Autodesk Fusion 360 part; units mm, degrees
(part 2 of 2)
  spline S369 degree 3 poles (-15.1942, 11.595) (-14.4543, 12.2873) (-14.1797, 12.9796) (-14.2633, 13.9224) knots 0 0 0 0 1 1 1 1
  spline S370 degree 3 poles (-14.2633, 13.9224) (-14.3946, 15.3547) (-15.6001, 16.4289) (-17.092, 16.4289) knots 0 0 0 0 1 1 1 1
  spline S371 degree 3 poles (-17.092, 16.4289) (-17.6291, 16.4289) (-18.7749, 15.7844) (-19.0733, 15.3189) knots 0 0 0 0 1 1 1 1
  spline S372 degree 3 poles (-19.0733, 15.3189) (-20.1355, 13.6837) (-19.4433, 11.6309) (-17.641, 11.058) knots 0 0 0 0 1 1 1 1
  spline S373 degree 3 poles (-17.641, 11.058) (-16.7403, 10.8043) (-15.715, 11.0847) (-15.1942, 11.595) knots 0 0 0 0 1 1 1 1
  spline S374 degree 3 poles (-66.0987, 20.2601) (-65.6691, 20.8688) (-65.5974, 21.4298) (-65.8361, 22.3369) knots 0 0 0 0 1 1 1 1
  spline S375 degree 3 poles (-65.8361, 22.3369) (-66.2061, 23.805) (-66.9461, 27.6482) (-67.161, 29.3191) knots 0 0 0 0 1 1 1 1
  spline S376 degree 3 poles (-67.161, 29.3191) (-67.2923, 30.2859) (-67.4474, 30.632) (-67.7577, 30.632) knots 0 0 0 0 1 1 1 1
  spline S377 degree 3 poles (-67.7577, 30.632) (-68.4142, 30.632) (-69.2497, 29.4265) (-69.2497, 28.4717) knots 0 0 0 0 1 1 1 1
  spline S378 degree 3 poles (-69.2497, 28.4717) (-69.2497, 27.9107) (-68.7364, 24.4733) (-68.5335, 23.5901) knots 0 0 0 0 1 1 1 1
  spline S379 degree 3 poles (-68.5335, 23.5901) (-68.3426, 22.8024) (-67.9368, 21.2388) (-67.7458, 20.5108) knots 0 0 0 0 1 1 1 1
  spline S380 degree 3 poles (-67.7458, 20.5108) (-67.6503, 20.1647) (-67.4594, 19.7708) (-67.3281, 19.6395) knots 0 0 0 0 1 1 1 1
  spline S381 degree 3 poles (-67.3281, 19.6395) (-67.1013, 19.4127) (-67.0774, 19.4127) (-66.7671, 19.5918) knots 0 0 0 0 1 1 1 1
  spline S382 degree 3 poles (-66.7671, 19.5918) (-66.5881, 19.6992) (-66.2897, 19.9976) (-66.0987, 20.2601) knots 0 0 0 0 1 1 1 1
  spline S383 degree 3 poles (-58.9494, 26.2159) (-58.0185, 26.3591) (-57.6127, 26.5978) (-57.4336, 27.123) knots 0 0 0 0 1 1 1 1
  spline S384 degree 3 poles (-57.4336, 27.123) (-57.171, 27.8988) (-57.5291, 28.2688) (-59.3314, 29.0685) knots 0 0 0 0 1 1 1 1
  spline S385 degree 3 poles (-59.3314, 29.0685) (-60.6084, 29.6294) (-60.9426, 29.6652) (-61.4917, 29.2833) knots 0 0 0 0 1 1 1 1
  spline S386 degree 3 poles (-61.4917, 29.2833) (-62.0884, 28.8894) (-62.351, 28.4478) (-62.4226, 27.7794) knots 0 0 0 0 1 1 1 1
  spline S387 degree 3 poles (-62.4226, 27.7794) (-62.4823, 27.0753) (-62.16, 26.4307) (-61.6349, 26.2278) knots 0 0 0 0 1 1 1 1
  spline S388 degree 3 poles (-61.6349, 26.2278) (-61.2171, 26.0727) (-59.9639, 26.0727) (-58.9494, 26.2159) knots 0 0 0 0 1 1 1 1
  spline S389 degree 3 poles (-19.3597, 26.3353) (-15.8984, 26.4427) (-15.0868, 26.5501) (-13.4159, 27.123) knots 0 0 0 0 1 1 1 1
  spline S390 degree 3 poles (-13.4159, 27.123) (-5.6927, 30.0385) (-15.6264, 35.7741) (-17.5933, 36.9697) knots 0 0 0 0 1 1 1 1
  spline S391 degree 3 poles (-17.5933, 36.9697) (-17.8678, 37.1487) (-19.8371, 38.3542) (-21.9497, 39.6552) knots 0 0 0 0 1 1 1 1
  spline S392 degree 3 poles (-21.9497, 39.6552) (-24.0742, 40.9681) (-26.0793, 42.1974) (-26.4255, 42.4003) knots 0 0 0 0 1 1 1 1
  spline S393 degree 3 poles (-26.4255, 42.4003) (-26.7716, 42.6032) (-28.0725, 43.379) (-29.3019, 44.1309) knots 0 0 0 0 1 1 1 1
  spline S394 degree 3 poles (-29.3019, 44.1309) (-30.5312, 44.8829) (-31.7725, 45.6229) (-32.047, 45.778) knots 0 0 0 0 1 1 1 1
  spline S395 degree 3 poles (-32.047, 45.778) (-32.6557, 46.1122) (-33.6464, 46.6851) (-35.5441, 47.7951) knots 0 0 0 0 1 1 1 1
  spline S396 degree 3 poles (-35.5441, 47.7951) (-38.3745, 49.7231) (-42.4002, 49.8932) (-44.7821, 48.2009) knots 0 0 0 0 1 1 1 1
  spline S397 degree 3 poles (-44.7821, 48.2009) (-45.6415, 47.5683) (-48.1837, 44.8709) (-50.2127, 42.4361) knots 0 0 0 0 1 1 1 1
  spline S398 degree 3 poles (-50.2127, 42.4361) (-50.7617, 41.7677) (-52.6714, 39.2016) (-53.3756, 38.1513) knots 0 0 0 0 1 1 1 1
  spline S399 degree 3 poles (-53.3756, 38.1513) (-53.8053, 37.5307) (-54.1753, 36.9936) (-54.2111, 36.9578) knots 0 0 0 0 1 1 1 1
  spline S400 degree 3 poles (-54.2111, 36.9578) (-54.2469, 36.922) (-54.3424, 36.7668) (-54.4378, 36.5997) knots 0 0 0 0 1 1 1 1
  spline S401 degree 3 poles (-54.4378, 36.5997) (-54.5333, 36.4326) (-54.8436, 35.8955) (-55.1301, 35.4062) knots 0 0 0 0 1 1 1 1
  spline S402 degree 3 poles (-55.1301, 35.4062) (-55.9536, 33.95) (-56.073, 32.673) (-55.512, 31.2049) knots 0 0 0 0 1 1 1 1
  spline S403 degree 3 poles (-55.512, 31.2049) (-54.7243, 29.1281) (-52.5759, 28.0778) (-48.0047, 27.5407) knots 0 0 0 0 1 1 1 1
  spline S404 degree 3 poles (-48.0047, 27.5407) (-39.6499, 26.562) (-27.9413, 26.0607) (-19.3597, 26.3353) knots 0 0 0 0 1 1 1 1
  spline S405 degree 3 poles (-63.9742, 31.2407) (-63.3655, 31.563) (-62.8046, 32.4343) (-62.7807, 33.1026) knots 0 0 0 0 1 1 1 1
  spline S406 degree 3 poles (-62.7807, 33.1026) (-62.7568, 33.4607) (-62.9597, 39.1181) (-63.0791, 41.6723) knots 0 0 0 0 1 1 1 1
  spline S407 degree 3 poles (-63.0791, 41.6723) (-63.1029, 42.0781) (-63.1507, 42.1616) (-63.3775, 42.1855) knots 0 0 0 0 1 1 1 1
  spline S408 degree 3 poles (-63.3775, 42.1855) (-63.9384, 42.269) (-64.8216, 41.4097) (-65.0842, 40.5265) knots 0 0 0 0 1 1 1 1
  spline S409 degree 3 poles (-65.0842, 40.5265) (-65.4303, 39.3568) (-65.3349, 35.3465) (-64.8813, 32.6133) knots 0 0 0 0 1 1 1 1
  spline S410 degree 3 poles (-64.8813, 32.6133) (-64.6307, 31.1214) (-64.5113, 30.9543) (-63.9742, 31.2407) knots 0 0 0 0 1 1 1 1
  spline S411 degree 3 poles (-59.1046, 34.9287) (-58.8539, 34.9287) (-58.2691, 35.7284) (-58.1617, 36.2416) knots 0 0 0 0 1 1 1 1
  spline S412 degree 3 poles (-58.1617, 36.2416) (-58.102, 36.54) (-58.0185, 37.7574) (-57.9707, 38.9629) knots 0 0 0 0 1 1 1 1
  spline S413 degree 3 poles (-57.9707, 38.9629) (-55.0055, 52.9367) (-60.0287, 51.9617) (-60.0594, 39.8939) knots 0 0 0 0 1 1 1 1
  spline S414 degree 3 poles (-60.0594, 39.8939) (-60.0475, 35.6091) (-59.9162, 34.6662) (-59.3672, 34.8691) knots 0 0 0 0 1 1 1 1
  spline S415 degree 3 poles (-59.3672, 34.8691) (-59.2717, 34.9049) (-59.1523, 34.9287) (-59.1046, 34.9287) knots 0 0 0 0 1 1 1 1
  spline S416 degree 3 poles (-53.483, 42.8897) (-53.0295, 43.1642) (-52.8504, 43.6535) (-52.5401, 45.4916) knots 0 0 0 0 1 1 1 1
  spline S417 degree 3 poles (-52.5401, 45.4916) (-47.8194, 56.8739) (-51.9428, 63.1533) (-54.1514, 48.6187) knots 0 0 0 0 1 1 1 1
  spline S418 degree 3 poles (-54.1514, 48.6187) (-54.4975, 46.3032) (-54.7004, 43.3551) (-54.5572, 42.9493) knots 0 0 0 0 1 1 1 1
  spline S419 degree 3 poles (-54.5572, 42.9493) (-54.4378, 42.6271) (-53.9843, 42.6032) (-53.483, 42.8897) knots 0 0 0 0 1 1 1 1
sketch "Sketch3" plane through (0, 0, 0) normal (0, 1, 0) x (1, 0, 0)
  circle A0 centre (-16.9405, 13.7) radius 2.65
  line L0 (-24.8905, 7.37) -> (-22.6383, 9.3908)
  line L1 (-24.4945, 12.3026) -> (-27.2771, 11.1137)
  arc A1 (-27.2771, 11.1137) -> (-24.8905, 7.37) centre (-26.3931, 9.0447) ccw
  arc A2 (-22.6383, 9.3908) -> (-24.4945, 12.3026) centre (-23.807, 10.6933) ccw
  line L2 (-60.0053, 29.4008) -> (-57.9336, 28.3794)
  line L3 (-60.4832, 26.1063) -> (-58.2067, 26.4969)
  arc A3 (-58.2067, 26.4969) -> (-57.9336, 28.3794) centre (-58.3758, 27.4825) ccw
  arc A4 (-60.0053, 29.4008) -> (-60.4832, 26.1063) centre (-60.7791, 27.8311) ccw
  line L4 (-66.9923, 29.5599) -> (-65.485, 21.1385)
  line L5 (-69.4532, 29.1195) -> (-67.9459, 20.698)
  line L6 (-63.025, 16.5893) -> (-64.9793, 2.8727)
  line L7 (-58.3449, -1.6991) -> (-24.4432, 17.0672)
  line L8 (-25.5471, 21.7521) -> (-55.2793, 23.0246)
  arc A5 (-24.4432, 17.0672) -> (-25.5471, 21.7521) centre (-25.654, 19.2544) ccw
  arc A6 (-55.2793, 23.0246) -> (-63.025, 16.5893) centre (-55.6, 15.5314) ccw
  arc A7 (-64.9793, 2.8727) -> (-58.3449, -1.6991) centre (-60.5243, 2.2379) ccw
  arc A8 (-66.9923, 29.5599) -> (-69.4532, 29.1195) centre (-68.2228, 29.3397) ccw
  arc A9 (-67.9459, 20.698) -> (-65.485, 21.1385) centre (-66.7155, 20.9182) ccw
  line L9 (-14.8187, 9.7316) -> (-21.3854, 6.2205)
  line L10 (-18.1944, 18.2109) -> (-16.902, 18.1998)
  arc A10 (-14.8187, 9.7316) -> (-16.902, 18.1998) centre (-16.9405, 13.7) ccw
  line L11 (-59.106, -8.2167) -> (-32.5692, 5.579)
  line L12 (-29.2713, 2.0763) -> (-49.4618, -31.6353)
  line L13 (-57.5245, -30.9331) -> (-62.6501, -17.5544)
  line L14 (-70.8774, 23.2307) -> (-66.9031, 10.8336)
  line L15 (-73.2581, 22.4675) -> (-69.2838, 10.0704)
  line L16 (-68.0088, 1.6737) -> (-73.8434, 13.4497)
  line L17 (-76.0835, 12.3397) -> (-70.2489, 0.5638)
  line L18 (-74.8007, 3.5823) -> (-70.4064, -3.84)
  line L19 (-72.5576, -5.1137) -> (-76.9519, 2.3086)
  line L20 (-15.8372, -7.9675) -> (-16.0798, -15.41)
  arc A11 (-15.8372, -7.9675) -> (-24.2125, -5.5377) centre (-20.3348, -7.8209) ccw
  circle A12 centre (-20.3348, -7.8209) radius 2.65
  line L21 (-18.8278, -17.8708) -> (-19.4518, -14.9099)
  arc A13 (-19.4518, -14.9099) -> (-22.9016, -15.0616) centre (-21.1642, -15.2708) ccw
  line L22 (-22.9016, -15.0616) -> (-23.2633, -18.0658)
  arc A14 (-23.2633, -18.0658) -> (-18.8278, -17.8708) centre (-21.0294, -18.3348) ccw
  line L23 (-27.701, -51.3778) -> (-27.0022, -12.6349)
  arc A15 (-27.0022, -12.6349) -> (-31.6114, -11.2483) centre (-29.5018, -12.5898) ccw
  line L24 (-31.6114, -11.2483) -> (-47.5795, -36.361)
  arc A16 (-47.5795, -36.361) -> (-45.8793, -46.2866) centre (-41.2506, -40.3853) ccw
  line L25 (-45.8793, -46.2866) -> (-34.9774, -54.8374)
  arc A17 (-34.9774, -54.8374) -> (-27.701, -51.3778) centre (-32.2002, -51.2966) ccw
  line L26 (-1.0185, -17.6992) -> (5.3056, -21.6305)
  arc A18 (-1.0185, -17.6992) -> (-7.3105, -23.7375) centre (-3.3943, -21.5209) ccw
  circle A19 centre (-3.3943, -21.5209) radius 2.65
  line L27 (6.0627, -25.2408) -> (3.1865, -24.3007)
  arc A20 (3.1865, -24.3007) -> (1.5929, -27.3642) centre (2.6428, -25.9641) ccw
  line L28 (1.5929, -27.3642) -> (4.0138, -29.1795)
  arc A21 (4.0138, -29.1795) -> (6.0627, -25.2408) centre (5.3637, -27.3794) ccw
  line L29 (30.644, -49.6786) -> (-2.559, -29.702)
  arc A22 (-2.559, -29.702) -> (-6.0644, -33.0005) centre (-3.8478, -31.8442) ccw
  line L30 (-6.0644, -33.0005) -> (7.6998, -59.3856)
  arc A23 (7.6998, -59.3856) -> (17.1457, -62.8759) centre (14.3494, -55.9167) ccw
  line L31 (17.1457, -62.8759) -> (30.0019, -57.7101)
  arc A24 (30.0019, -57.7101) -> (30.644, -49.6786) centre (28.3241, -53.5345) ccw
  line L32 (14.8187, -9.7316) -> (21.3854, -6.2205)
  arc A25 (14.8187, -9.7316) -> (16.902, -18.1998) centre (16.9405, -13.7) ccw
  circle A26 centre (16.9405, -13.7) radius 2.65
  line L33 (24.8905, -7.37) -> (22.6383, -9.3908)
  arc A27 (22.6383, -9.3908) -> (24.4945, -12.3026) centre (23.807, -10.6933) ccw
  line L34 (24.4945, -12.3026) -> (27.2771, -11.1137)
  arc A28 (27.2771, -11.1137) -> (24.8905, -7.37) centre (26.3931, -9.0447) ccw
  line L35 (58.3449, 1.6991) -> (24.4432, -17.0672)
  arc A29 (24.4432, -17.0672) -> (25.5471, -21.7521) centre (25.654, -19.2544) ccw
  line L36 (25.5471, -21.7521) -> (55.2793, -23.0246)
  arc A30 (55.2793, -23.0246) -> (63.025, -16.5893) centre (55.6, -15.5314) ccw
  line L37 (63.025, -16.5893) -> (64.9793, -2.8727)
  arc A31 (64.9793, -2.8727) -> (58.3449, 1.6991) centre (60.5243, -2.2379) ccw
  line L38 (15.8372, 7.9675) -> (16.0798, 15.41)
  arc A32 (15.8372, 7.9675) -> (24.2125, 5.5377) centre (20.3348, 7.8209) ccw
  circle A33 centre (20.3348, 7.8209) radius 2.65
  line L39 (18.8278, 17.8708) -> (19.4518, 14.9099)
  arc A34 (19.4518, 14.9099) -> (22.9016, 15.0616) centre (21.1642, 15.2708) ccw
  line L40 (22.9016, 15.0616) -> (23.2633, 18.0658)
  arc A35 (23.2633, 18.0658) -> (18.8278, 17.8708) centre (21.0294, 18.3348) ccw
  line L41 (27.701, 51.3778) -> (27.0022, 12.6349)
  arc A36 (27.0022, 12.6349) -> (31.6114, 11.2483) centre (29.5018, 12.5898) ccw
  line L42 (31.6114, 11.2483) -> (47.5795, 36.361)
  arc A37 (47.5795, 36.361) -> (45.8793, 46.2866) centre (41.2506, 40.3853) ccw
  line L43 (45.8793, 46.2866) -> (34.9774, 54.8374)
  arc A38 (34.9774, 54.8374) -> (27.701, 51.3778) centre (32.2002, 51.2966) ccw
  line L44 (1.0185, 17.6992) -> (-5.3056, 21.6305)
  arc A39 (1.0185, 17.6992) -> (7.3105, 23.7375) centre (3.3943, 21.5209) ccw
  circle A40 centre (3.3943, 21.5209) radius 2.65
  line L45 (-6.0627, 25.2408) -> (-3.1865, 24.3007)
  arc A41 (-3.1865, 24.3007) -> (-1.5929, 27.3642) centre (-2.6428, 25.9641) ccw
  line L46 (-1.5929, 27.3642) -> (-4.0138, 29.1795)
  arc A42 (-4.0138, 29.1795) -> (-6.0627, 25.2408) centre (-5.3637, 27.3794) ccw
  line L47 (-30.644, 49.6786) -> (2.559, 29.702)
  arc A43 (2.559, 29.702) -> (6.0644, 33.0005) centre (3.8478, 31.8442) ccw
  line L48 (6.0644, 33.0005) -> (-7.6998, 59.3856)
  arc A44 (-7.6998, 59.3856) -> (-17.1457, 62.8759) centre (-14.3494, 55.9167) ccw
  line L49 (-17.1457, 62.8759) -> (-30.0019, 57.7101)
  arc A45 (-30.0019, 57.7101) -> (-30.644, 49.6786) centre (-28.3241, 53.5345) ccw
  arc A46 (-29.2713, 2.0763) -> (-32.5692, 5.579) centre (-31.4161, 3.3609) ccw
  arc A47 (-59.106, -8.2167) -> (-62.6501, -17.5544) centre (-55.6465, -14.8712) ccw
  arc A48 (-57.5245, -30.9331) -> (-49.4618, -31.6353) centre (-53.3224, -29.3232) ccw
  line L50 (-16.4338, -24.3115) -> (2.6661, -58.6528)
  arc A49 (-16.4338, -24.3115) -> (-21.1162, -25.4163) centre (-18.6186, -25.5267) ccw
  line L51 (-22.4371, -55.2957) -> (-21.1162, -25.4163)
  arc A50 (-22.4371, -55.2957) -> (-16.1225, -63.0338) centre (-14.9444, -55.6269) ccw
  line L52 (-1.9734, -65.2842) -> (-16.1225, -63.0338)
  arc A51 (-1.9734, -65.2842) -> (2.6661, -58.6528) centre (-1.2666, -60.8401) ccw
  line L53 (12.8375, -26.3878) -> (52.1279, -27.0175)
  arc A52 (12.8375, -26.3878) -> (11.453, -30.9953) centre (12.7974, -28.8875) ccw
  line L54 (36.6689, -47.0789) -> (11.453, -30.9953)
  arc A53 (36.6689, -47.0789) -> (46.5276, -45.4794) centre (40.7021, -40.7557) ccw
  line L55 (55.5511, -34.3512) -> (46.5276, -45.4794)
  arc A54 (55.5511, -34.3512) -> (52.1279, -27.0175) centre (52.0558, -31.5169) ccw
  line L56 (29.2713, -2.0763) -> (49.4618, 31.6353)
  arc A55 (29.2713, -2.0763) -> (32.5692, -5.579) centre (31.4161, -3.3609) ccw
  line L57 (59.106, 8.2167) -> (32.5692, -5.579)
  arc A56 (59.106, 8.2167) -> (62.6501, 17.5544) centre (55.6465, 14.8712) ccw
  line L58 (57.5245, 30.9331) -> (62.6501, 17.5544)
  arc A57 (57.5245, 30.9331) -> (49.4618, 31.6353) centre (53.3224, 29.3232) ccw
  line L59 (16.4338, 24.3115) -> (-2.6661, 58.6528)
  arc A58 (16.4338, 24.3115) -> (21.1162, 25.4163) centre (18.6186, 25.5267) ccw
  line L60 (22.4371, 55.2957) -> (21.1162, 25.4163)
  arc A59 (22.4371, 55.2957) -> (16.1225, 63.0338) centre (14.9444, 55.6269) ccw
  line L61 (1.9734, 65.2842) -> (16.1225, 63.0338)
  arc A60 (1.9734, 65.2842) -> (-2.6661, 58.6528) centre (1.2666, 60.8401) ccw
  line L62 (-12.8375, 26.3878) -> (-52.1279, 27.0175)
  arc A61 (-12.8375, 26.3878) -> (-11.453, 30.9953) centre (-12.7974, 28.8875) ccw
  line L63 (-36.6689, 47.0789) -> (-11.453, 30.9953)
  arc A62 (-36.6689, 47.0789) -> (-46.5276, 45.4794) centre (-40.7021, 40.7557) ccw
  line L64 (-55.5511, 34.3512) -> (-46.5276, 45.4794)
  arc A63 (-55.5511, 34.3512) -> (-52.1279, 27.0175) centre (-52.0558, 31.5169) ccw
  arc A64 (-70.8774, 23.2307) -> (-73.2581, 22.4675) centre (-72.0677, 22.8491) ccw
  arc A65 (-69.2838, 10.0704) -> (-66.9031, 10.8336) centre (-68.0934, 10.452) ccw
  arc A66 (-70.2489, 0.5638) -> (-68.0088, 1.6737) centre (-69.1288, 1.1187) ccw
  arc A67 (-73.8434, 13.4497) -> (-76.0835, 12.3397) centre (-74.9634, 12.8947) ccw
  arc A68 (-74.8007, 3.5823) -> (-76.9519, 2.3086) centre (-75.8763, 2.9454) ccw
  arc A69 (-72.5576, -5.1137) -> (-70.4064, -3.84) centre (-71.482, -4.4769) ccw
  line L65 (-18.3054, 22.707) -> (-11.1638, 23.121)
  line L66 (-28.8175, -4.4994) -> (-25.6053, 1.8924)
  line L67 (-10.5122, -27.2064) -> (-14.4415, -21.2286)
  line L68 (18.3054, -22.707) -> (11.1638, -23.121)
  line L69 (28.8175, 4.4994) -> (25.6053, -1.8924)
  line L70 (10.5122, 27.2064) -> (14.4415, 21.2286)
  line L71 (-24.8683, -6.6514) -> (-24.2125, -5.5377)
  line L72 (-6.6739, -24.8622) -> (-7.3105, -23.7375)
  line L73 (18.1944, -18.2109) -> (16.902, -18.1998)
  line L74 (24.8683, 6.6514) -> (24.2125, 5.5377)
  line L75 (6.6739, 24.8622) -> (7.3105, 23.7375)
  arc A70 (-18.3054, 22.707) -> (-18.1944, 18.2109) centre (-18.1752, 20.4608) ccw
  arc A71 (-5.3056, 21.6305) -> (-11.1638, 23.121) centre (-10.5851, 13.1378) ccw
  arc A72 (10.5122, 27.2064) -> (6.6739, 24.8622) centre (8.632, 25.9705) ccw
  arc A73 (16.0798, 15.41) -> (14.4415, 21.2286) centre (6.0851, 15.7358) ccw
  arc A74 (21.3854, -6.2205) -> (25.6053, -1.8924) centre (16.6702, 2.5981) ccw
  arc A75 (28.8175, 4.4994) -> (24.8683, 6.6514) centre (26.8071, 5.5098) ccw
  arc A76 (5.3056, -21.6305) -> (11.1638, -23.121) centre (10.5851, -13.1378) ccw
  arc A77 (18.3054, -22.707) -> (18.1944, -18.2109) centre (18.1752, -20.4608) ccw
  arc A78 (-16.0798, -15.41) -> (-14.4415, -21.2286) centre (-6.0851, -15.7358) ccw
  arc A79 (-10.5122, -27.2064) -> (-6.6739, -24.8622) centre (-8.632, -25.9705) ccw
  arc A80 (-21.3854, 6.2205) -> (-25.6053, 1.8924) centre (-16.6702, -2.5981) ccw
  arc A81 (-15.9874, -12.5747) -> (-15.5594, -12.5362) centre (-16.6702, -2.5981) ccw
  arc A82 (-28.8175, -4.4994) -> (-24.8683, -6.6514) centre (-26.8071, -5.5098) ccw
  line L76 (-66.6665, -4.5408) -> (-64.3617, -4.3895)
  arc A83 (-66.6665, -4.5408) -> (-65.4331, -7.6328) centre (-66.5518, -6.2871) ccw
  arc A84 (-63.6569, -6.1563) -> (-64.3617, -4.3895) centre (-64.2961, -5.3873) ccw
  line L77 (-65.4331, -7.6328) -> (-63.6569, -6.1563)
  arc A85 (-69.1919, -16.048) -> (-67.2809, -14.4361) centre (-68.2364, -15.242) ccw
  line L78 (-74.708, -9.5084) -> (-69.1919, -16.048)
  arc A86 (-72.797, -7.8965) -> (-74.708, -9.5084) centre (-73.7525, -8.7025) ccw
  line L79 (-72.797, -7.8965) -> (-67.2809, -14.4361)
  arc A87 (-65.0367, -25.9207) -> (-63.3566, -24.0694) centre (-64.1966, -24.9951) ccw
  line L80 (-74.6771, -17.1716) -> (-65.0367, -25.9207)
  arc A88 (-72.997, -15.3203) -> (-74.6771, -17.1716) centre (-73.837, -16.246) ccw
  line L81 (-72.997, -15.3203) -> (-63.3566, -24.0694)
  line L82 (-72.0601, -27.3552) -> (-61.1192, -34.6362)
  arc A89 (-61.1192, -34.6362) -> (-59.7342, -32.5549) centre (-60.4267, -33.5956) ccw
  arc A90 (-70.6751, -25.2739) -> (-72.0601, -27.3552) centre (-71.3676, -26.3146) ccw
  line L83 (-59.7342, -32.5549) -> (-70.6751, -25.2739)
  arc A91 (-60.2799, -40.7074) -> (-59.0537, -38.5288) centre (-59.6668, -39.6181) ccw
  line L84 (-60.2799, -40.7074) -> (-67.7966, -36.4766)
  arc A92 (-66.5704, -34.298) -> (-67.7966, -36.4766) centre (-67.1835, -35.3873) ccw
  line L85 (-66.5704, -34.298) -> (-59.0537, -38.5288)
  line L86 (-55.4644, -37.2657) -> (-53.5441, -35.9822)
  arc A93 (-55.4644, -37.2657) -> (-52.8503, -39.3268) centre (-54.492, -38.7207) ccw
  arc A94 (-52.0503, -37.16) -> (-53.5441, -35.9822) centre (-52.9884, -36.8136) ccw
  line L87 (-52.8503, -39.3268) -> (-52.0503, -37.16)
  arc A95 (-51.8979, -48.4939) -> (-51.0489, -46.1425) centre (-51.4734, -47.3182) ccw
  line L88 (-59.9448, -45.5885) -> (-51.8979, -48.4939)
  arc A96 (-59.0958, -43.2371) -> (-59.9448, -45.5885) centre (-59.5203, -44.4128) ccw
  line L89 (-59.0958, -43.2371) -> (-51.0489, -46.1425)
  arc A97 (-43.3631, -54.9663) -> (-42.8337, -52.523) centre (-43.0984, -53.7447) ccw
  line L90 (-56.0865, -52.2096) -> (-43.3631, -54.9663)
  arc A98 (-55.5571, -49.7663) -> (-56.0865, -52.2096) centre (-55.8218, -50.9879) ccw
  line L91 (-55.5571, -49.7663) -> (-42.8337, -52.523)
  line L92 (-48.7283, -59.7204) -> (-35.6127, -60.5554)
  arc A99 (-35.6127, -60.5554) -> (-35.4538, -58.0605) centre (-35.5333, -59.308) ccw
  arc A100 (-48.5694, -57.2254) -> (-48.7283, -59.7204) centre (-48.6489, -58.4729) ccw
  line L93 (-35.4538, -58.0605) -> (-48.5694, -57.2254)
  arc A101 (-31.8503, -65.3936) -> (-31.8776, -62.8937) centre (-31.8639, -64.1437) ccw
  line L94 (-31.8503, -65.3936) -> (-40.4753, -65.488)
  arc A102 (-40.5027, -62.9882) -> (-40.4753, -65.488) centre (-40.489, -64.2381) ccw
  line L95 (-40.5027, -62.9882) -> (-31.8776, -62.8937)
  line L96 (-29.4008, -60.0053) -> (-28.3794, -57.9336)
  arc A103 (-29.4008, -60.0053) -> (-26.1063, -60.4832) centre (-27.8311, -60.7791) ccw
  arc A104 (-26.4969, -58.2067) -> (-28.3794, -57.9336) centre (-27.4825, -58.3758) ccw
  line L97 (-26.1063, -60.4832) -> (-26.4969, -58.2067)
  arc A105 (-20.698, -67.9459) -> (-21.1385, -65.485) centre (-20.9182, -66.7155) ccw
  line L98 (-29.1195, -69.4532) -> (-20.698, -67.9459)
  arc A106 (-29.5599, -66.9923) -> (-29.1195, -69.4532) centre (-29.3397, -68.2228) ccw
  line L99 (-29.5599, -66.9923) -> (-21.1385, -65.485)
  arc A107 (-10.0704, -69.2838) -> (-10.8336, -66.9031) centre (-10.452, -68.0934) ccw
  line L100 (-22.4675, -73.2581) -> (-10.0704, -69.2838)
  arc A108 (-23.2307, -70.8774) -> (-22.4675, -73.2581) centre (-22.8491, -72.0677) ccw
  line L101 (-23.2307, -70.8774) -> (-10.8336, -66.9031)
  line L102 (-12.3397, -76.0835) -> (-0.5638, -70.2489)
  arc A109 (-0.5638, -70.2489) -> (-1.6737, -68.0088) centre (-1.1187, -69.1288) ccw
  arc A110 (-13.4497, -73.8434) -> (-12.3397, -76.0835) centre (-12.8947, -74.9634) ccw
  line L103 (-1.6737, -68.0088) -> (-13.4497, -73.8434)
  arc A111 (5.1137, -72.5576) -> (3.84, -70.4064) centre (4.4769, -71.482) ccw
  line L104 (5.1137, -72.5576) -> (-2.3086, -76.9519)
  arc A112 (-3.5823, -74.8007) -> (-2.3086, -76.9519) centre (-2.9454, -75.8763) ccw
  line L105 (-3.5823, -74.8007) -> (3.84, -70.4064)
  line L106 (4.5408, -66.6665) -> (4.3895, -64.3617)
  arc A113 (4.5408, -66.6665) -> (7.6328, -65.4331) centre (6.2871, -66.5518) ccw
  arc A114 (6.1563, -63.6569) -> (4.3895, -64.3617) centre (5.3873, -64.2961) ccw
  line L107 (7.6328, -65.4331) -> (6.1563, -63.6569)
  arc A115 (16.048, -69.1919) -> (14.4361, -67.2809) centre (15.242, -68.2364) ccw
  line L108 (9.5084, -74.708) -> (16.048, -69.1919)
  arc A116 (7.8965, -72.797) -> (9.5084, -74.708) centre (8.7025, -73.7525) ccw
  line L109 (7.8965, -72.797) -> (14.4361, -67.2809)
  arc A117 (25.9207, -65.0367) -> (24.0694, -63.3566) centre (24.9951, -64.1966) ccw
  line L110 (17.1716, -74.6771) -> (25.9207, -65.0367)
  arc A118 (15.3203, -72.997) -> (17.1716, -74.6771) centre (16.246, -73.837) ccw
  line L111 (15.3203, -72.997) -> (24.0694, -63.3566)
  line L112 (27.3552, -72.0601) -> (34.6362, -61.1192)
  arc A119 (34.6362, -61.1192) -> (32.5549, -59.7342) centre (33.5956, -60.4267) ccw
  arc A120 (25.2739, -70.6751) -> (27.3552, -72.0601) centre (26.3146, -71.3676) ccw
  line L113 (32.5549, -59.7342) -> (25.2739, -70.6751)
  arc A121 (40.7074, -60.2799) -> (38.5288, -59.0537) centre (39.6181, -59.6668) ccw
  line L114 (40.7074, -60.2799) -> (36.4766, -67.7966)
  arc A122 (34.298, -66.5704) -> (36.4766, -67.7966) centre (35.3873, -67.1835) ccw
  line L115 (34.298, -66.5704) -> (38.5288, -59.0537)
  line L116 (37.2657, -55.4644) -> (35.9822, -53.5441)
  arc A123 (37.2657, -55.4644) -> (39.3268, -52.8503) centre (38.7207, -54.492) ccw
  arc A124 (37.16, -52.0503) -> (35.9822, -53.5441) centre (36.8136, -52.9884) ccw
  line L117 (39.3268, -52.8503) -> (37.16, -52.0503)
  arc A125 (48.4939, -51.8979) -> (46.1425, -51.0489) centre (47.3182, -51.4734) ccw
  line L118 (45.5885, -59.9448) -> (48.4939, -51.8979)
  arc A126 (43.2371, -59.0958) -> (45.5885, -59.9448) centre (44.4128, -59.5203) ccw
  line L119 (43.2371, -59.0958) -> (46.1425, -51.0489)
  arc A127 (54.9663, -43.3631) -> (52.523, -42.8337) centre (53.7447, -43.0984) ccw
  line L120 (52.2096, -56.0865) -> (54.9663, -43.3631)
  arc A128 (49.7663, -55.5571) -> (52.2096, -56.0865) centre (50.9879, -55.8218) ccw
  line L121 (49.7663, -55.5571) -> (52.523, -42.8337)
  line L122 (59.7204, -48.7283) -> (60.5554, -35.6127)
  arc A129 (60.5554, -35.6127) -> (58.0605, -35.4538) centre (59.308, -35.5333) ccw
  arc A130 (57.2254, -48.5694) -> (59.7204, -48.7283) centre (58.4729, -48.6489) ccw
  line L123 (58.0605, -35.4538) -> (57.2254, -48.5694)
  arc A131 (65.3936, -31.8503) -> (62.8937, -31.8776) centre (64.1437, -31.8639) ccw
  line L124 (65.3936, -31.8503) -> (65.488, -40.4753)
  arc A132 (62.9882, -40.5027) -> (65.488, -40.4753) centre (64.2381, -40.489) ccw
  line L125 (62.9882, -40.5027) -> (62.8937, -31.8776)
  line L126 (60.0053, -29.4008) -> (57.9336, -28.3794)
  arc A133 (60.0053, -29.4008) -> (60.4832, -26.1063) centre (60.7791, -27.8311) ccw
  arc A134 (58.2067, -26.4969) -> (57.9336, -28.3794) centre (58.3758, -27.4825) ccw
  line L127 (60.4832, -26.1063) -> (58.2067, -26.4969)
  arc A135 (67.9459, -20.698) -> (65.485, -21.1385) centre (66.7155, -20.9182) ccw
  line L128 (69.4532, -29.1195) -> (67.9459, -20.698)
  arc A136 (66.9923, -29.5599) -> (69.4532, -29.1195) centre (68.2228, -29.3397) ccw
  line L129 (66.9923, -29.5599) -> (65.485, -21.1385)
  arc A137 (69.2838, -10.0704) -> (66.9031, -10.8336) centre (68.0934, -10.452) ccw
  line L130 (73.2581, -22.4675) -> (69.2838, -10.0704)
  arc A138 (70.8774, -23.2307) -> (73.2581, -22.4675) centre (72.0677, -22.8491) ccw
  line L131 (70.8774, -23.2307) -> (66.9031, -10.8336)
  line L132 (76.0835, -12.3397) -> (70.2489, -0.5638)
  arc A139 (70.2489, -0.5638) -> (68.0088, -1.6737) centre (69.1288, -1.1187) ccw
  arc A140 (73.8434, -13.4497) -> (76.0835, -12.3397) centre (74.9634, -12.8947) ccw
  line L133 (68.0088, -1.6737) -> (73.8434, -13.4497)
  arc A141 (72.5576, 5.1137) -> (70.4064, 3.84) centre (71.482, 4.4769) ccw
  line L134 (72.5576, 5.1137) -> (76.9519, -2.3086)
  arc A142 (74.8007, -3.5823) -> (76.9519, -2.3086) centre (75.8763, -2.9454) ccw
  line L135 (74.8007, -3.5823) -> (70.4064, 3.84)
  line L136 (66.6665, 4.5408) -> (64.3617, 4.3895)
  arc A143 (66.6665, 4.5408) -> (65.4331, 7.6328) centre (66.5518, 6.2871) ccw
  arc A144 (63.6569, 6.1563) -> (64.3617, 4.3895) centre (64.2961, 5.3873) ccw
  line L137 (65.4331, 7.6328) -> (63.6569, 6.1563)
  arc A145 (69.1919, 16.048) -> (67.2809, 14.4361) centre (68.2364, 15.242) ccw
  line L138 (74.708, 9.5084) -> (69.1919, 16.048)
  arc A146 (72.797, 7.8965) -> (74.708, 9.5084) centre (73.7525, 8.7025) ccw
  line L139 (72.797, 7.8965) -> (67.2809, 14.4361)
  arc A147 (65.0367, 25.9207) -> (63.3566, 24.0694) centre (64.1966, 24.9951) ccw
  line L140 (74.6771, 17.1716) -> (65.0367, 25.9207)
  arc A148 (72.997, 15.3203) -> (74.6771, 17.1716) centre (73.837, 16.246) ccw
  line L141 (72.997, 15.3203) -> (63.3566, 24.0694)
  line L142 (72.0601, 27.3552) -> (61.1192, 34.6362)
  arc A149 (61.1192, 34.6362) -> (59.7342, 32.5549) centre (60.4267, 33.5956) ccw
  arc A150 (70.6751, 25.2739) -> (72.0601, 27.3552) centre (71.3676, 26.3146) ccw
  line L143 (59.7342, 32.5549) -> (70.6751, 25.2739)
  arc A151 (60.2799, 40.7074) -> (59.0537, 38.5288) centre (59.6668, 39.6181) ccw
  line L144 (60.2799, 40.7074) -> (67.7966, 36.4766)
  arc A152 (66.5704, 34.298) -> (67.7966, 36.4766) centre (67.1835, 35.3873) ccw
  line L145 (66.5704, 34.298) -> (59.0537, 38.5288)
  line L146 (55.4644, 37.2657) -> (53.5441, 35.9822)
  arc A153 (55.4644, 37.2657) -> (52.8503, 39.3268) centre (54.492, 38.7207) ccw
  arc A154 (52.0503, 37.16) -> (53.5441, 35.9822) centre (52.9884, 36.8136) ccw
  line L147 (52.8503, 39.3268) -> (52.0503, 37.16)
  arc A155 (51.8979, 48.4939) -> (51.0489, 46.1425) centre (51.4734, 47.3182) ccw
  line L148 (59.9448, 45.5885) -> (51.8979, 48.4939)
  arc A156 (59.0958, 43.2371) -> (59.9448, 45.5885) centre (59.5203, 44.4128) ccw
  line L149 (59.0958, 43.2371) -> (51.0489, 46.1425)
  arc A157 (43.3631, 54.9663) -> (42.8337, 52.523) centre (43.0984, 53.7447) ccw
  line L150 (56.0865, 52.2096) -> (43.3631, 54.9663)
  arc A158 (55.5571, 49.7663) -> (56.0865, 52.2096) centre (55.8218, 50.9879) ccw
  line L151 (55.5571, 49.7663) -> (42.8337, 52.523)
  line L152 (48.7283, 59.7204) -> (35.6127, 60.5554)
  arc A159 (35.6127, 60.5554) -> (35.4538, 58.0605) centre (35.5333, 59.308) ccw
  arc A160 (48.5694, 57.2254) -> (48.7283, 59.7204) centre (48.6489, 58.4729) ccw
  line L153 (35.4538, 58.0605) -> (48.5694, 57.2254)
  arc A161 (31.8503, 65.3936) -> (31.8776, 62.8937) centre (31.8639, 64.1437) ccw
  line L154 (31.8503, 65.3936) -> (40.4753, 65.488)
  arc A162 (40.5027, 62.9882) -> (40.4753, 65.488) centre (40.489, 64.2381) ccw
  line L155 (40.5027, 62.9882) -> (31.8776, 62.8937)
  line L156 (29.4008, 60.0053) -> (28.3794, 57.9336)
  arc A163 (29.4008, 60.0053) -> (26.1063, 60.4832) centre (27.8311, 60.7791) ccw
  arc A164 (26.4969, 58.2067) -> (28.3794, 57.9336) centre (27.4825, 58.3758) ccw
  line L157 (26.1063, 60.4832) -> (26.4969, 58.2067)
  arc A165 (20.698, 67.9459) -> (21.1385, 65.485) centre (20.9182, 66.7155) ccw
  line L158 (29.1195, 69.4532) -> (20.698, 67.9459)
  arc A166 (29.5599, 66.9923) -> (29.1195, 69.4532) centre (29.3397, 68.2228) ccw
  line L159 (29.5599, 66.9923) -> (21.1385, 65.485)
  arc A167 (10.0704, 69.2838) -> (10.8336, 66.9031) centre (10.452, 68.0934) ccw
  line L160 (22.4675, 73.2581) -> (10.0704, 69.2838)
  arc A168 (23.2307, 70.8774) -> (22.4675, 73.2581) centre (22.8491, 72.0677) ccw
  line L161 (23.2307, 70.8774) -> (10.8336, 66.9031)
  line L162 (12.3397, 76.0835) -> (0.5638, 70.2489)
  arc A169 (0.5638, 70.2489) -> (1.6737, 68.0088) centre (1.1187, 69.1288) ccw
  arc A170 (13.4497, 73.8434) -> (12.3397, 76.0835) centre (12.8947, 74.9634) ccw
  line L163 (1.6737, 68.0088) -> (13.4497, 73.8434)
  arc A171 (-5.1137, 72.5576) -> (-3.84, 70.4064) centre (-4.4769, 71.482) ccw
  line L164 (-5.1137, 72.5576) -> (2.3086, 76.9519)
  arc A172 (3.5823, 74.8007) -> (2.3086, 76.9519) centre (2.9454, 75.8763) ccw
  line L165 (3.5823, 74.8007) -> (-3.84, 70.4064)
  line L166 (-4.5408, 66.6665) -> (-4.3895, 64.3617)
  arc A173 (-4.5408, 66.6665) -> (-7.6328, 65.4331) centre (-6.2871, 66.5518) ccw
  arc A174 (-6.1563, 63.6569) -> (-4.3895, 64.3617) centre (-5.3873, 64.2961) ccw
  line L167 (-7.6328, 65.4331) -> (-6.1563, 63.6569)
  arc A175 (-16.048, 69.1919) -> (-14.4361, 67.2809) centre (-15.242, 68.2364) ccw
  line L168 (-9.5084, 74.708) -> (-16.048, 69.1919)
  arc A176 (-7.8965, 72.797) -> (-9.5084, 74.708) centre (-8.7025, 73.7525) ccw
  line L169 (-7.8965, 72.797) -> (-14.4361, 67.2809)
  arc A177 (-25.9207, 65.0367) -> (-24.0694, 63.3566) centre (-24.9951, 64.1966) ccw
  line L170 (-17.1716, 74.6771) -> (-25.9207, 65.0367)
  arc A178 (-15.3203, 72.997) -> (-17.1716, 74.6771) centre (-16.246, 73.837) ccw
  line L171 (-15.3203, 72.997) -> (-24.0694, 63.3566)
  line L172 (-27.3552, 72.0601) -> (-34.6362, 61.1192)
  arc A179 (-34.6362, 61.1192) -> (-32.5549, 59.7342) centre (-33.5956, 60.4267) ccw
  arc A180 (-25.2739, 70.6751) -> (-27.3552, 72.0601) centre (-26.3146, 71.3676) ccw
  line L173 (-32.5549, 59.7342) -> (-25.2739, 70.6751)
  arc A181 (-40.7074, 60.2799) -> (-38.5288, 59.0537) centre (-39.6181, 59.6668) ccw
  line L174 (-40.7074, 60.2799) -> (-36.4766, 67.7966)
  arc A182 (-34.298, 66.5704) -> (-36.4766, 67.7966) centre (-35.3873, 67.1835) ccw
  line L175 (-34.298, 66.5704) -> (-38.5288, 59.0537)
  line L176 (-37.2657, 55.4644) -> (-35.9822, 53.5441)
  arc A183 (-37.2657, 55.4644) -> (-39.3268, 52.8503) centre (-38.7207, 54.492) ccw
  arc A184 (-37.16, 52.0503) -> (-35.9822, 53.5441) centre (-36.8136, 52.9884) ccw
  line L177 (-39.3268, 52.8503) -> (-37.16, 52.0503)
  arc A185 (-48.4939, 51.8979) -> (-46.1425, 51.0489) centre (-47.3182, 51.4734) ccw
  line L178 (-45.5885, 59.9448) -> (-48.4939, 51.8979)
  arc A186 (-43.2371, 59.0958) -> (-45.5885, 59.9448) centre (-44.4128, 59.5203) ccw
  line L179 (-43.2371, 59.0958) -> (-46.1425, 51.0489)
  arc A187 (-54.9663, 43.3631) -> (-52.523, 42.8337) centre (-53.7447, 43.0984) ccw
  line L180 (-52.2096, 56.0865) -> (-54.9663, 43.3631)
  arc A188 (-49.7663, 55.5571) -> (-52.2096, 56.0865) centre (-50.9879, 55.8218) ccw
  line L181 (-49.7663, 55.5571) -> (-52.523, 42.8337)
  line L182 (-59.7204, 48.7283) -> (-60.5554, 35.6127)
  arc A189 (-60.5554, 35.6127) -> (-58.0605, 35.4538) centre (-59.308, 35.5333) ccw
  arc A190 (-57.2254, 48.5694) -> (-59.7204, 48.7283) centre (-58.4729, 48.6489) ccw
  line L183 (-58.0605, 35.4538) -> (-57.2254, 48.5694)
  arc A191 (-65.3936, 31.8503) -> (-62.8937, 31.8776) centre (-64.1437, 31.8639) ccw
  line L184 (-65.3936, 31.8503) -> (-65.488, 40.4753)
  arc A192 (-62.9882, 40.5027) -> (-65.488, 40.4753) centre (-64.2381, 40.489) ccw
  line L185 (-62.9882, 40.5027) -> (-62.8937, 31.8776)
  spline S0 degree 5 poles (-68.3276, 35.1404) (-68.4477, 34.8399) (-68.7325, 34.2029) (-69.293, 33.1393) (-70.2797, 31.5364) (-71.7515, 29.4037) (-73.2511, 27.3606) (-74.5616, 25.6154) (-75.4989, 24.2916) (-75.9632, 23.4101) (-75.9614, 22.7362) (-75.7035, 21.9554) (-75.5189, 21.0588) (-75.6798, 20.0399) (-76.1657, 18.6131) (-76.8308, 16.8879) (-77.4937, 15.2187) (-77.9796, 13.8724) (-78.1692, 13.0347) (-78.0803, 12.0717) (-77.8409, 10.7241) (-77.5915, 9.6554) (-77.4758, 9.398) (-77.6659, 8.9103) (-78.1499, 7.5307) (-78.7561, 5.5413) (-79.253, 3.436) (-79.4215, 1.7592) (-79.1255, 0.6372) (-78.4191, -0.4269) (-77.5582, -1.5197) (-76.9991, -2.4276) (-76.7789, -3.0913) (-76.7378, -3.5203) (-76.7436, -3.7313) knots 0 0 0 0 0 0 0.033333 0.066667 0.1 0.133333 0.166667 0.2 0.233333 0.266667 0.3 0.333333 0.366667 0.4 0.433333 0.466667 0.5 0.533333 0.566667 0.6 0.633333 0.666667 0.7 0.733333 0.766667 0.8 0.833333 0.866667 0.9 0.933333 0.966667 1 1 1 1 1 1
  line L186 (-66.2839, 40.2512) -> (-70.3713, 30.0296)
  line L187 (-75.2102, 26.4622) -> (-76.5585, 20.1817)
  line L188 (-74.5849, 26.4682) -> (-76.7403, 14.2994)
  line L189 (-77.8362, 17.9795) -> (-78.3674, 7.9864)
  line L190 (-77.6115, 11.6792) -> (-77.4834, 7.1908)
  line L191 (-76.5928, 1.7021) -> (-76.8944, -9.1648)
  line L192 (-80.2252, 7.6378) -> (-78.3068, -4.6783)
  spline S1 degree 5 poles (-76.7436, -3.7313) (-76.9031, -4.463) (-77.2012, -5.8758) (-77.5857, -7.8431) (-77.9729, -10.1621) (-78.2487, -12.5567) (-78.3211, -14.4606) (-78.2019, -15.9056) (-77.912, -16.9479) (-77.485, -17.6776) (-76.969, -18.2227) (-76.4322, -18.7643) (-75.9443, -19.488) (-75.5569, -20.5291) (-75.2778, -21.9069) (-75.0655, -23.5074) (-74.8549, -25.1538) (-74.5761, -26.6552) (-74.1755, -27.8651) (-73.6366, -28.7346) (-73.0013, -29.3709) (-72.3416, -29.9643) (-71.7318, -30.716) (-71.2172, -31.7586) (-70.7928, -33.1003) (-70.4206, -34.6679) (-70.0413, -36.3334) (-69.5879, -37.9475) (-68.9976, -39.3681) (-68.227, -40.4957) (-67.2519, -41.2747) (-66.299, -41.5974) (-65.4859, -41.6672) (-64.9001, -41.6373) (-64.5962, -41.6032) knots 0 0 0 0 0 0 0.033333 0.066667 0.1 0.133333 0.166667 0.2 0.233333 0.266667 0.3 0.333333 0.366667 0.4 0.433333 0.466667 0.5 0.533333 0.566667 0.6 0.633333 0.666667 0.7 0.733333 0.766667 0.8 0.833333 0.866667 0.9 0.933333 0.966667 1 1 1 1 1 1
  spline S2 degree 5 poles (-64.5962, -41.6032) (-64.3685, -42.3166) (-63.9203, -43.6892) (-63.2697, -45.5852) (-62.4455, -47.7871) (-61.487, -49.9988) (-60.5978, -51.6838) (-59.772, -52.8756) (-58.9998, -53.6333) (-58.2652, -54.0517) (-57.5458, -54.2658) (-56.8101, -54.4665) (-56.0257, -54.8493) (-55.1696, -55.5572) (-54.239, -56.6108) (-53.2549, -57.8908) (-52.2494, -59.2112) (-51.2572, -60.3721) (-50.3053, -61.2197) (-49.4039, -61.7032) (-48.5355, -61.9365) (-47.6675, -62.1206) (-46.7636, -62.4668) (-45.7966, -63.1124) (-44.7582, -64.0621) (-43.652, -65.2336) (-42.4908, -66.4862) (-41.2911, -67.6575) (-40.0696, -68.5925) (-38.8385, -69.1838) (-37.6045, -69.3709) (-36.6179, -69.174) (-35.8788, -68.8278) (-35.3865, -68.509) (-35.1404, -68.3276) knots 0 0 0 0 0 0 0.033333 0.066667 0.1 0.133333 0.166667 0.2 0.233333 0.266667 0.3 0.333333 0.366667 0.4 0.433333 0.466667 0.5 0.533333 0.566667 0.6 0.633333 0.666667 0.7 0.733333 0.766667 0.8 0.833333 0.866667 0.9 0.933333 0.966667 1 1 1 1 1 1
  spline S3 degree 5 poles (-35.1404, -68.3276) (-34.5865, -68.8315) (-33.512, -69.7961) (-32.0005, -71.1128) (-30.1858, -72.6076) (-28.2499, -74.0437) (-26.6373, -75.0584) (-25.3263, -75.6776) (-24.2786, -75.9477) (-23.4333, -75.9428) (-22.7032, -75.7685) (-21.9657, -75.5744) (-21.0951, -75.5137) (-19.9997, -75.6987) (-18.6669, -76.1459) (-17.1747, -76.7623) (-15.6437, -77.4031) (-14.204, -77.9123) (-12.9558, -78.1705) (-11.9334, -78.1385) (-11.0647, -77.9064) (-10.221, -77.6318) (-9.265, -77.4796) (-8.1048, -77.5552) (-6.7306, -77.8585) (-5.187, -78.32) (-3.555, -78.8242) (-1.9304, -79.2386) (-0.4051, -79.4377) (0.9568, -79.3342) (2.119, -78.8792) (2.8749, -78.2154) (3.3419, -77.546) (3.6089, -77.0238) (3.7313, -76.7436) knots 0 0 0 0 0 0 0.033333 0.066667 0.1 0.133333 0.166667 0.2 0.233333 0.266667 0.3 0.333333 0.366667 0.4 0.433333 0.466667 0.5 0.533333 0.566667 0.6 0.633333 0.666667 0.7 0.733333 0.766667 0.8 0.833333 0.866667 0.9 0.933333 0.966667 1 1 1 1 1 1
  spline S4 degree 5 poles (3.7313, -76.7436) (4.463, -76.9031) (5.8758, -77.2012) (7.8431, -77.5857) (10.1621, -77.9729) (12.5567, -78.2487) (14.4606, -78.3211) (15.9056, -78.2019) (16.9479, -77.912) (17.6776, -77.485) (18.2227, -76.969) (18.7643, -76.4322) (19.488, -75.9443) (20.5291, -75.5569) (21.9069, -75.2778) (23.5074, -75.0655) (25.1538, -74.8549) (26.6552, -74.5761) (27.8651, -74.1755) (28.7346, -73.6366) (29.3709, -73.0013) (29.9643, -72.3416) (30.716, -71.7318) (31.7586, -71.2172) (33.1003, -70.7928) (34.6679, -70.4206) (36.3334, -70.0413) (37.9475, -69.5879) (39.3681, -68.9976) (40.4957, -68.227) (41.2747, -67.2519) (41.5974, -66.299) (41.6672, -65.4859) (41.6373, -64.9001) (41.6032, -64.5962) knots 0 0 0 0 0 0 0.033333 0.066667 0.1 0.133333 0.166667 0.2 0.233333 0.266667 0.3 0.333333 0.366667 0.4 0.433333 0.466667 0.5 0.533333 0.566667 0.6 0.633333 0.666667 0.7 0.733333 0.766667 0.8 0.833333 0.866667 0.9 0.933333 0.966667 1 1 1 1 1 1
  spline S5 degree 5 poles (41.6032, -64.5962) (42.3166, -64.3685) (43.6892, -63.9203) (45.5852, -63.2697) (47.7871, -62.4455) (49.9988, -61.487) (51.6838, -60.5978) (52.8756, -59.772) (53.6333, -58.9998) (54.0517, -58.2652) (54.2658, -57.5458) (54.4665, -56.8101) (54.8493, -56.0257) (55.5572, -55.1696) (56.6108, -54.239) (57.8908, -53.2549) (59.2112, -52.2494) (60.3721, -51.2572) (61.2197, -50.3053) (61.7032, -49.4039) (61.9365, -48.5355) (62.1206, -47.6675) (62.4668, -46.7636) (63.1124, -45.7966) (64.0621, -44.7582) (65.2336, -43.652) (66.4862, -42.4908) (67.6575, -41.2911) (68.5925, -40.0696) (69.1838, -38.8385) (69.3709, -37.6045) (69.174, -36.6179) (68.8278, -35.8788) (68.509, -35.3865) (68.3276, -35.1404) knots 0 0 0 0 0 0 0.033333 0.066667 0.1 0.133333 0.166667 0.2 0.233333 0.266667 0.3 0.333333 0.366667 0.4 0.433333 0.466667 0.5 0.533333 0.566667 0.6 0.633333 0.666667 0.7 0.733333 0.766667 0.8 0.833333 0.866667 0.9 0.933333 0.966667 1 1 1 1 1 1
  spline S6 degree 5 poles (68.3276, -35.1404) (68.8315, -34.5865) (69.7961, -33.512) (71.1128, -32.0005) (72.6076, -30.1858) (74.0437, -28.2499) (75.0584, -26.6373) (75.6776, -25.3263) (75.9477, -24.2786) (75.9428, -23.4333) (75.7685, -22.7032) (75.5744, -21.9657) (75.5137, -21.0951) (75.6987, -19.9997) (76.1459, -18.6669) (76.7623, -17.1747) (77.4031, -15.6437) (77.9123, -14.204) (78.1705, -12.9558) (78.1385, -11.9334) (77.9064, -11.0647) (77.6318, -10.221) (77.4796, -9.265) (77.5552, -8.1048) (77.8585, -6.7306) (78.32, -5.187) (78.8242, -3.555) (79.2386, -1.9304) (79.4377, -0.4051) (79.3342, 0.9568) (78.8792, 2.119) (78.2154, 2.8749) (77.546, 3.3419) (77.0238, 3.6089) (76.7436, 3.7313) knots 0 0 0 0 0 0 0.033333 0.066667 0.1 0.133333 0.166667 0.2 0.233333 0.266667 0.3 0.333333 0.366667 0.4 0.433333 0.466667 0.5 0.533333 0.566667 0.6 0.633333 0.666667 0.7 0.733333 0.766667 0.8 0.833333 0.866667 0.9 0.933333 0.966667 1 1 1 1 1 1
  spline S7 degree 5 poles (76.7436, 3.7313) (76.9031, 4.463) (77.2012, 5.8758) (77.5857, 7.8431) (77.9729, 10.1621) (78.2487, 12.5567) (78.3211, 14.4606) (78.2019, 15.9056) (77.912, 16.9479) (77.485, 17.6776) (76.969, 18.2227) (76.4322, 18.7643) (75.9443, 19.488) (75.5569, 20.5291) (75.2778, 21.9069) (75.0655, 23.5074) (74.8549, 25.1538) (74.5761, 26.6552) (74.1755, 27.8651) (73.6366, 28.7346) (73.0013, 29.3709) (72.3416, 29.9643) (71.7318, 30.716) (71.2172, 31.7586) (70.7928, 33.1003) (70.4206, 34.6679) (70.0413, 36.3334) (69.5879, 37.9475) (68.9976, 39.3681) (68.227, 40.4957) (67.2519, 41.2747) (66.299, 41.5974) (65.4859, 41.6672) (64.9001, 41.6373) (64.5962, 41.6032) knots 0 0 0 0 0 0 0.033333 0.066667 0.1 0.133333 0.166667 0.2 0.233333 0.266667 0.3 0.333333 0.366667 0.4 0.433333 0.466667 0.5 0.533333 0.566667 0.6 0.633333 0.666667 0.7 0.733333 0.766667 0.8 0.833333 0.866667 0.9 0.933333 0.966667 1 1 1 1 1 1
  spline S8 degree 5 poles (64.5962, 41.6032) (64.3685, 42.3166) (63.9203, 43.6892) (63.2697, 45.5852) (62.4455, 47.7871) (61.487, 49.9988) (60.5978, 51.6838) (59.772, 52.8756) (58.9998, 53.6333) (58.2652, 54.0517) (57.5458, 54.2658) (56.8101, 54.4665) (56.0257, 54.8493) (55.1696, 55.5572) (54.239, 56.6108) (53.2549, 57.8908) (52.2494, 59.2112) (51.2572, 60.3721) (50.3053, 61.2197) (49.4039, 61.7032) (48.5355, 61.9365) (47.6675, 62.1206) (46.7636, 62.4668) (45.7966, 63.1124) (44.7582, 64.0621) (43.652, 65.2336) (42.4908, 66.4862) (41.2911, 67.6575) (40.0696, 68.5925) (38.8385, 69.1838) (37.6045, 69.3709) (36.6179, 69.174) (35.8788, 68.8278) (35.3865, 68.509) (35.1404, 68.3276) knots 0 0 0 0 0 0 0.033333 0.066667 0.1 0.133333 0.166667 0.2 0.233333 0.266667 0.3 0.333333 0.366667 0.4 0.433333 0.466667 0.5 0.533333 0.566667 0.6 0.633333 0.666667 0.7 0.733333 0.766667 0.8 0.833333 0.866667 0.9 0.933333 0.966667 1 1 1 1 1 1
  spline S9 degree 5 poles (35.1404, 68.3276) (34.5865, 68.8315) (33.512, 69.7961) (32.0005, 71.1128) (30.1858, 72.6076) (28.2499, 74.0437) (26.6373, 75.0584) (25.3263, 75.6776) (24.2786, 75.9477) (23.4333, 75.9428) (22.7032, 75.7685) (21.9657, 75.5744) (21.0951, 75.5137) (19.9997, 75.6987) (18.6669, 76.1459) (17.1747, 76.7623) (15.6437, 77.4031) (14.204, 77.9123) (12.9558, 78.1705) (11.9334, 78.1385) (11.0647, 77.9064) (10.221, 77.6318) (9.265, 77.4796) (8.1048, 77.5552) (6.7306, 77.8585) (5.187, 78.32) (3.555, 78.8242) (1.9304, 79.2386) (0.4051, 79.4377) (-0.9568, 79.3342) (-2.119, 78.8792) (-2.8749, 78.2154) (-3.3419, 77.546) (-3.6089, 77.0238) (-3.7313, 76.7436) knots 0 0 0 0 0 0 0.033333 0.066667 0.1 0.133333 0.166667 0.2 0.233333 0.266667 0.3 0.333333 0.366667 0.4 0.433333 0.466667 0.5 0.533333 0.566667 0.6 0.633333 0.666667 0.7 0.733333 0.766667 0.8 0.833333 0.866667 0.9 0.933333 0.966667 1 1 1 1 1 1
  spline S10 degree 5 poles (-3.7313, 76.7436) (-4.463, 76.9031) (-5.8758, 77.2012) (-7.8431, 77.5857) (-10.1621, 77.9729) (-12.5567, 78.2487) (-14.4606, 78.3211) (-15.9056, 78.2019) (-16.9479, 77.912) (-17.6776, 77.485) (-18.2227, 76.969) (-18.7643, 76.4322) (-19.488, 75.9443) (-20.5291, 75.5569) (-21.9069, 75.2778) (-23.5074, 75.0655) (-25.1538, 74.8549) (-26.6552, 74.5761) (-27.8651, 74.1755) (-28.7346, 73.6366) (-29.3709, 73.0013) (-29.9643, 72.3416) (-30.716, 71.7318) (-31.7586, 71.2172) (-33.1003, 70.7928) (-34.6679, 70.4206) (-36.3334, 70.0413) (-37.9475, 69.5879) (-39.3681, 68.9976) (-40.4957, 68.227) (-41.2747, 67.2519) (-41.5974, 66.299) (-41.6672, 65.4859) (-41.6373, 64.9001) (-41.6032, 64.5962) knots 0 0 0 0 0 0 0.033333 0.066667 0.1 0.133333 0.166667 0.2 0.233333 0.266667 0.3 0.333333 0.366667 0.4 0.433333 0.466667 0.5 0.533333 0.566667 0.6 0.633333 0.666667 0.7 0.733333 0.766667 0.8 0.833333 0.866667 0.9 0.933333 0.966667 1 1 1 1 1 1
  spline S11 degree 5 poles (-41.6032, 64.5962) (-42.3166, 64.3685) (-43.6892, 63.9203) (-45.5852, 63.2697) (-47.7871, 62.4455) (-49.9988, 61.487) (-51.6838, 60.5978) (-52.8756, 59.772) (-53.6333, 58.9998) (-54.0517, 58.2652) (-54.2658, 57.5458) (-54.4665, 56.8101) (-54.8493, 56.0257) (-55.5572, 55.1696) (-56.6108, 54.239) (-57.8908, 53.2549) (-59.2112, 52.2494) (-60.3721, 51.2572) (-61.2197, 50.3053) (-61.7032, 49.4039) (-61.9365, 48.5355) (-62.1206, 47.6675) (-62.4668, 46.7636) (-63.1124, 45.7966) (-64.0621, 44.7582) (-65.2336, 43.652) (-66.4862, 42.4908) (-67.6575, 41.2911) (-68.5925, 40.0696) (-69.1838, 38.8385) (-69.3709, 37.6045) (-69.174, 36.6179) (-68.8278, 35.8788) (-68.509, 35.3865) (-68.3276, 35.1404) knots 0 0 0 0 0 0 0.033333 0.066667 0.1 0.133333 0.166667 0.2 0.233333 0.266667 0.3 0.333333 0.366667 0.4 0.433333 0.466667 0.5 0.533333 0.566667 0.6 0.633333 0.666667 0.7 0.733333 0.766667 0.8 0.833333 0.866667 0.9 0.933333 0.966667 1 1 1 1 1 1
  point P0 (-52.8503, -39.3268)
  point P1 (7.6328, -65.4331)
  point P2 (60.4832, -26.1063)
  point P3 (52.8503, 39.3268)
  point P4 (-7.6328, 65.4331)
  point P5 (-75.8843, 23.3219)
  point P6 (-75.6626, 20.3838)
  point P7 (-78.1018, 12.9829)
  point P8 (-77.5475, 9.435)
  point P9 (-79.266, 1.4797)
  point P10 (-77.3787, -17.7448)
  point P11 (-75.7176, -20.1784)
  point P12 (-74.1296, -27.8074)
  point P13 (-71.8755, -30.6028)
  point P14 (-69.3862, -38.3515)
  point P15 (-58.1396, -54.0568)
  point P16 (-55.4842, -55.3338)
  point P17 (-50.2945, -61.1467)
  point P18 (-46.9446, -62.4406)
  point P19 (-40.9145, -67.9065)
  point P20 (-23.3219, -75.8843)
  point P21 (-20.3838, -75.6626)
  point P22 (-12.9829, -78.1018)
  point P23 (-9.435, -77.5475)
  point P24 (-1.4797, -79.266)
  point P25 (17.7448, -77.3787)
  point P26 (20.1784, -75.7176)
  point P27 (27.8074, -74.1296)
  point P28 (30.6028, -71.8755)
  point P29 (38.3515, -69.3862)
  point P30 (54.0568, -58.1396)
  point P31 (55.3338, -55.4842)
  point P32 (61.1467, -50.2945)
  point P33 (62.4406, -46.9446)
  point P34 (67.9065, -40.9145)
  point P35 (75.8843, -23.3219)
  point P36 (75.6626, -20.3838)
  point P37 (78.1018, -12.9829)
  point P38 (77.5475, -9.435)
  point P39 (79.266, -1.4797)
  point P40 (77.3787, 17.7448)
  point P41 (75.7176, 20.1784)
  point P42 (74.1296, 27.8074)
  point P43 (71.8755, 30.6028)
  point P44 (69.3862, 38.3515)
  point P45 (58.1396, 54.0568)
  point P46 (55.4842, 55.3338)
  point P47 (50.2945, 61.1467)
  point P48 (46.9446, 62.4406)
  point P49 (40.9145, 67.9065)
  point P50 (23.3219, 75.8843)
  point P51 (20.3838, 75.6626)
  point P52 (12.9829, 78.1018)
  point P53 (9.435, 77.5475)
  point P54 (1.4797, 79.266)
  point P55 (-17.7448, 77.3787)
  point P56 (-20.1784, 75.7176)
  point P57 (-27.8074, 74.1296)
  point P58 (-30.6028, 71.8755)
  point P59 (-38.3515, 69.3862)
  point P60 (-54.0568, 58.1396)
  point P61 (-55.3338, 55.4842)
  point P62 (-61.1467, 50.2945)
  point P63 (-62.4406, 46.9446)
  point P64 (-67.9065, 40.9145)
  dimension "d3" = 5.3
  dimension "d4" = 3.5
  dimension "d5" = 4.5
  dimension "d6" = 4.5
  dimension "d7" = 15
  dimension "d8" = 9
  dimension "d9" = 20
  dimension "d10" = 9
  dimension "d11" = 2
  dimension "d12" = 3.5
  dimension "d13" = 2.5
  dimension "d14" = 2.5
  dimension "d15" = 5
  dimension "d16" = 5
  dimension "d17" = 15
  dimension "d18" = 9
  dimension "d19" = 2.5
  dimension "d20" = 2.5
  dimension "d21" = 2.5
  dimension "d22" = 2.5
  dimension "d23" = 2.5
  dimension "d24" = 2.5
  dimension "d28" = 360
  constraint coincident A0.centre A10.centre
  constraint tangent L0 A2
  constraint tangent L0 A1
  constraint tangent L1 A2
  constraint tangent L1 A1
  constraint tangent L2 A3
  constraint tangent L2 A4
  constraint tangent L3 A3
  constraint tangent L3 A4
  constraint tangent L4 A9
  constraint tangent L5 A9
  constraint tangent L4 A8
  constraint tangent L5 A8
  constraint tangent L8 A5
  constraint tangent L8 A6
  constraint tangent L6 A6
  constraint tangent L6 A7
  constraint tangent L7 A7
  constraint tangent L7 A5
  constraint tangent L9 A10
  constraint tangent L9 A80
  constraint tangent L10 A10
  constraint tangent L10 A70
  constraint tangent L11 A47
  constraint tangent L11 A46
  constraint tangent L12 A48
  constraint tangent L12 A46
  constraint tangent L13 A48
  constraint tangent L13 A47
  constraint tangent L14 A65
  constraint tangent L15 A65
  constraint tangent L14 A64
  constraint tangent L15 A64
  constraint tangent L16 A67
  constraint tangent L17 A66
  constraint tangent L16 A66
  constraint tangent L17 A67
  constraint tangent L18 A69
  constraint tangent L19 A68
  constraint tangent L18 A68
  constraint tangent L19 A69
  constraint tangent L65 A70
  constraint coincident L20 A81.start
  constraint concentric A80 A81
  constraint midpoint S0.start L186
  constraint midpoint P5 L187
  constraint midpoint P6 L188
  constraint midpoint P7 L189
  constraint midpoint P8 L190
  constraint midpoint S0.end L191
  constraint coincident L19 L191.start
  constraint midpoint P9 L192
  constraint coincident S0.start S11.end
  measures "d3" diameter of A0
  measures "d4" diameter of A2
  measures "d5" diameter of A1
  measures "d6" diameter of A70
  measures "d7" diameter of A6
  measures "d8" diameter of A7
  measures "d9" diameter of A80
  measures "d10" diameter of A10
  measures "d11" diameter of A3
  measures "d12" diameter of A4
  measures "d13" diameter of A8
  measures "d14" diameter of A9
  measures "d15" diameter of A5
  measures "d16" diameter of A46
  measures "d17" diameter of A47
  measures "d18" diameter of A48
  measures "d19" diameter of A64
  measures "d20" diameter of A65
  measures "d21" diameter of A66
  measures "d22" diameter of A67
  measures "d23" diameter of A68
  measures "d24" diameter of A69
extrude "Extrude1" add sketch "Sketch3" along normal blind 1.7
equation "d2 = 38.5 mm + 5.3 mm"
